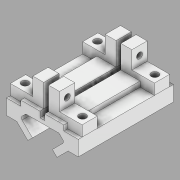
# Autodesk Inventor part: carriage
Saved by Autodesk Inventor 2020 (Build 240168000, 168)
## iProperties
Created: 2021-04-01
Part Number: carriage
Material: ABS Plastic
Document SubType Name: Modeling
Designer: griss
Density: 1.06 g/cm^3
Appearance: Smooth - White
Mass: 192.23 g
Surface Area: 415.711 cm^2
Volume: 181.35 cm^3
Author: griss
Autodesk Inventor part; units mm, degrees
sketch "Sketch1" plane through (0, 0, 0) normal (0, 0, 1) x (1, 0, 0)
  line L0 (0, 17.9605) -> (17.9605, 0) construction
  line L1 (17.9605, 0) -> (0, -17.9605) construction
  line L2 (0, -17.9605) -> (-17.9605, 0) construction
  line L3 (-17.9605, 0) -> (0, 17.9605) construction
  line L4 (0, 17.9605) -> (0, -17.9605) construction
  line L5 (17.9605, 0) -> (-17.9605, 0) construction
  line L6 (0, -30.115) -> (0, 54.9665) projected
  line L7 (-27.2882, 23.4644) -> (-11.7319, 7.908) construction
  line L8 (-11.7319, 7.908) -> (-6.7821, 12.8578) construction
  line L9 (-6.7821, 12.8578) -> (-22.3385, 28.4141) construction
  line L10 (-27.2882, 23.4644) -> (-22.3385, 28.4141) construction
  line L11 (27.2882, 23.4644) -> (11.7319, 7.908) construction
  line L12 (11.7319, 7.908) -> (6.7821, 12.8578) construction
  line L13 (6.7821, 12.8578) -> (22.3385, 28.4141) construction
  line L14 (27.2882, 23.4644) -> (22.3385, 28.4141) construction
  line L15 (-13.3307, 6.837) -> (-29.3711, 22.8773)
  line L16 (-29.3711, 22.8773) -> (-22.2034, 30.045)
  line L17 (-22.2034, 30.045) -> (0, 30.045)
  line L18 (-47.8625, 35.7423) -> (-28.7516, 35.7423)
  line L19 (-28.7516, 35.7423) -> (-28.7516, 42.812)
  line L20 (-28.7516, 42.812) -> (0, 42.812)
  line L21 (-47.8625, 15.4627) -> (-47.8625, 35.7423)
  line L22 (-47.8625, 15.4627) -> (-34.2195, 15.4627)
  line L23 (-34.2195, 15.4627) -> (-19.4622, 0.7055)
  line L24 (-19.4622, 0.7055) -> (-13.3307, 6.837)
  line L25 (13.3307, 6.837) -> (29.3711, 22.8773)
  line L26 (29.3711, 22.8773) -> (22.2034, 30.045)
  line L27 (22.2034, 30.045) -> (0, 30.045)
  line L28 (47.8625, 35.7423) -> (28.7516, 35.7423)
  line L29 (28.7516, 35.7423) -> (28.7516, 42.812)
  line L30 (28.7516, 42.812) -> (0, 42.812)
  line L31 (47.8625, 15.4627) -> (47.8625, 35.7423)
  line L32 (47.8625, 15.4627) -> (34.2195, 15.4627)
  line L33 (34.2195, 15.4627) -> (19.4622, 0.7055)
  line L34 (19.4622, 0.7055) -> (13.3307, 6.837)
  point P0 (0, 0)
  point P1 (0, 0)
  point P2 (0, 0)
  point P3 (0, 0)
  dimension "d2" = 25.4
  dimension "d3" = 25.4
  dimension "d6" = 22
  dimension "d14" = 7
  constraints: 68 end point, 14 horizontal alignment, 6 perpendicular, 4 midpoint, 3 horizontal, 2 coincident, 2 parallel, 1 vertical, 3 other
  measures "d2" distance of L1.end L2.end
  measures "d3" distance of L0.end L1.end
  measures "d6" distance of L8.end L9.end
  measures "d14" distance of L7.end L8.end
extrude "Carriage Frame" add sketch "Sketch1" along normal mid plane 127
fillet "Fillet1" radius 3.175 4 edges at (-29.3711, 22.8773, 0) (-22.2034, 30.045, 0) (22.2034, 30.045, 0) (29.3711, 22.8773, 0)
sketch "Sketch7" plane through (-47.8625, 35.7423, -63.5) normal (0, 1, 0) x (1, 0, 0)
  line L0 (19.1109, 0) -> (76.6141, 0) projected
  line L1 (19.1109, 0) -> (19.1109, -127) projected
  line L2 (76.6141, -127) -> (19.1109, -127) projected
  line L3 (76.6141, 0) -> (76.6141, -127) projected
  line L4 (0, 0) -> (19.1109, 0) projected
  line L5 (0, 0) -> (0, -127) projected
  line L6 (19.1109, -127) -> (0, -127) projected
  line L7 (19.1109, 0) -> (19.1109, -127) projected
  line L8 (76.6141, 0) -> (95.725, 0) projected
  line L9 (76.6141, 0) -> (76.6141, -127) projected
  line L10 (95.725, -127) -> (76.6141, -127) projected
  line L11 (95.725, -127) -> (95.725, 0) projected
  line L12 (19.1109, -63.5) -> (76.6141, -63.5) construction
  line L13 (47.8625, -63.5) -> (47.8625, -63.5) construction
  line L14 (16.8262, -19.4378) -> (9.5554, -23.6355)
  line L15 (9.5554, -23.6355) -> (2.2847, -19.4378)
  line L16 (2.2847, -19.4378) -> (2.2847, -11.0422)
  line L17 (2.2847, -11.0422) -> (9.5554, -6.8445)
  line L18 (9.5554, -6.8445) -> (16.8262, -11.0422)
  line L19 (16.8262, -11.0422) -> (16.8262, -19.4378)
  line L20 (78.8988, -19.4378) -> (86.1695, -23.6355)
  line L21 (86.1695, -23.6355) -> (93.4403, -19.4378)
  line L22 (93.4403, -19.4378) -> (93.4403, -11.0422)
  line L23 (93.4403, -11.0422) -> (86.1695, -6.8445)
  line L24 (86.1695, -6.8445) -> (78.8988, -11.0422)
  line L25 (78.8988, -11.0422) -> (78.8988, -19.4378)
  line L26 (16.8262, -107.5622) -> (9.5554, -103.3645)
  line L27 (9.5554, -103.3645) -> (2.2847, -107.5622)
  line L28 (2.2847, -107.5622) -> (2.2847, -115.9578)
  line L29 (2.2847, -115.9578) -> (9.5554, -120.1555)
  line L30 (9.5554, -120.1555) -> (16.8262, -115.9578)
  line L31 (16.8262, -115.9578) -> (16.8262, -107.5622)
  line L32 (78.8988, -115.9578) -> (78.8988, -107.5622)
  line L33 (86.1695, -120.1555) -> (78.8988, -115.9578)
  line L34 (78.8988, -107.5622) -> (86.1695, -103.3645)
  line L35 (93.4403, -115.9578) -> (86.1695, -120.1555)
  line L36 (93.4403, -107.5622) -> (93.4403, -115.9578)
  line L37 (86.1695, -103.3645) -> (93.4403, -107.5622)
  circle A0 centre (9.5554, -15.24) radius 4.8006
  circle A1 centre (86.1695, -15.24) radius 4.8006
  circle A2 centre (9.5554, -111.76) radius 4.8006
  circle A3 centre (86.1695, -111.76) radius 4.8006
  point P0 (9.5554, 0)
  dimension "d61" = 15.24
  dimension "d78" = 14.5415
  dimension "d79" = 9.6012
  constraints: 52 end point, 27 symmetric about line, 5 coincident, 4 centre point, 4 midpoint, 1 vertical, 1 vertical alignment, 16 other
  measures "d61" distance from line of L4 point (9.555, -15.24)
  measures "d78" distance between parallel lines of L19 L16
  measures "d79" diameter of A0
extrude "Carriage Screw" cut sketch "Sketch7" against normal through all contours A0 | A1 | A2 | A3
extrude "Carriage Screw Insert" cut sketch "Sketch7" against normal blind 6.35 contours L14 L15 L16 L17 L18 L19 | L25 L24 L23 L22 L21 L20 | L31 L30 L29 L28 L27 L26 | L32 L34 L37 L36 L35 L33 | A3
sketch "Ball Bearings" plane through (-13.3307, 6.837, -63.5) normal (0.7071, 0.7071, 0) x (-0.7071, 0.7071, 0)
  line L0 (19.5095, 127) -> (19.5095, 0) projected
  line L1 (0, 127) -> (19.5095, 127) projected
  line L2 (0, 0) -> (0, 127) projected
  line L3 (19.5095, 0) -> (0, 0) projected
  circle A0 centre (7.62, 96.52) radius 4
  line L4 (19.5095, 63.5) -> (0, 63.5) construction
  circle A1 centre (7.62, 30.48) radius 4
  point P0 (-14.2607, 63.5)
  dimension "d94" = 8
  dimension "d106" = 33.02
  dimension "d107" = 7.62
  constraints: 2 centre point, 2 end point, 2 midpoint, 1 symmetric about line, 1 other
  measures "d94" diameter of A0
  measures "d106" distance from line of L4 A0.centre
  measures "d107" distance from line of L2 A0.centre
ref_plane "Carriage Mid Plane" through (0, 15.4627, -63.5) normal (-1, 0, 0) x (0, 0, 1)
extrude "Ball Bearing Hole" cut sketch "Ball Bearings" against normal up to surface (8.6713 mm away) contours A0 | A1
mirror "Mirror4" about plane through (0, 15.4627, -63.5) normal (-1, 0, 0) of "Ball Bearing Hole"
sketch "Sketch13" plane through (0, 0, 63.5) normal (0, 0, 1) x (1, 0, 0)
  line L0 (47.8625, 35.7423) -> (28.7516, 35.7423) projected
  line L1 (28.7516, 35.7423) -> (28.7516, 42.812) projected
  line L2 (28.7516, 42.812) -> (-28.7516, 42.812) projected
  line L3 (-28.7516, 42.812) -> (-28.7516, 35.7423) projected
  line L4 (-28.7516, 35.7423) -> (-47.8625, 35.7423) projected
  line L5 (-47.8625, 35.7423) -> (-47.8625, 15.4627) projected
  line L6 (-47.8625, 15.4627) -> (-34.2195, 15.4627) projected
  line L7 (-34.2195, 15.4627) -> (-19.4622, 0.7055) projected
  line L8 (-19.4622, 0.7055) -> (-13.3307, 6.837) projected
  line L9 (-13.3307, 6.837) -> (-27.126, 20.6323) projected
  arc A0 (-27.126, 25.1224) -> (-27.126, 20.6323) centre (-24.8809, 22.8773) ccw projected
  line L10 (-27.126, 25.1224) -> (-23.1333, 29.1151) projected
  arc A1 (-20.8883, 30.045) -> (-23.1333, 29.1151) centre (-20.8883, 26.87) ccw projected
  line L11 (-20.8883, 30.045) -> (20.8883, 30.045) projected
  arc A2 (23.1333, 29.1151) -> (20.8883, 30.045) centre (20.8883, 26.87) ccw projected
  line L12 (23.1333, 29.1151) -> (27.126, 25.1224) projected
  arc A3 (27.126, 20.6323) -> (27.126, 25.1224) centre (24.8809, 22.8773) ccw projected
  line L13 (27.126, 20.6323) -> (13.3307, 6.837) projected
  line L14 (13.3307, 6.837) -> (19.4622, 0.7055) projected
  line L15 (19.4622, 0.7055) -> (34.2195, 15.4627) projected
  line L16 (34.2195, 15.4627) -> (47.8625, 15.4627) projected
  line L17 (47.8625, 15.4627) -> (47.8625, 35.7423) projected
  line L18 (-3.175, 42.812) -> (3.175, 42.812)
  line L19 (3.175, 42.812) -> (3.175, 35.1375)
  line L20 (3.175, 35.1375) -> (-3.175, 35.1375)
  line L21 (-3.175, 35.1375) -> (-3.175, 42.812)
  point P0 (0, 0)
  point P1 (0, 42.812)
  point P2 (0, 42.812)
  dimension "d112" = 6.35
  constraints: 8 end point, 2 midpoint, 2 parallel, 1 coincident, 1 horizontal, 1 perpendicular, 1 point on line
  measures "d112" distance of L19.end L20.end
extrude "Extrusion11" cut sketch "Sketch13" against normal up to surface (127 mm away) contours L19 L20 L21 L2
ref_plane "Work Plane3" through (0, 0, 48.26) normal (0, 0, 1) x (1, 0, 0)
sketch "Sketch15" plane through (0, 0, 48.26) normal (0, 0, 1) x (1, 0, 0)
  line L0 (-3.175, 35.1375) -> (-3.175, 42.812) projected
  line L1 (-3.175, 42.812) -> (-28.7516, 42.812) projected
  line L2 (-28.7516, 42.812) -> (-28.7516, 35.7423) projected
  line L3 (-28.7516, 35.7423) -> (-47.8625, 35.7423) projected
  line L4 (-47.8625, 35.7423) -> (-47.8625, 15.4627) projected
  line L5 (-47.8625, 15.4627) -> (-34.2195, 15.4627) projected
  line L6 (-34.2195, 15.4627) -> (-19.4622, 0.7055) projected
  line L7 (-19.4622, 0.7055) -> (-13.3307, 6.837) projected
  line L8 (-13.3307, 6.837) -> (-27.126, 20.6323) projected
  arc A0 (-27.126, 25.1224) -> (-27.126, 20.6323) centre (-24.8809, 22.8773) ccw projected
  line L9 (-27.126, 25.1224) -> (-23.1333, 29.1151) projected
  arc A1 (-20.8883, 30.045) -> (-23.1333, 29.1151) centre (-20.8883, 26.87) ccw projected
  line L10 (-20.8883, 30.045) -> (20.8883, 30.045) projected
  arc A2 (23.1333, 29.1151) -> (20.8883, 30.045) centre (20.8883, 26.87) ccw projected
  line L11 (23.1333, 29.1151) -> (27.126, 25.1224) projected
  arc A3 (27.126, 20.6323) -> (27.126, 25.1224) centre (24.8809, 22.8773) ccw projected
  line L12 (27.126, 20.6323) -> (13.3307, 6.837) projected
  line L13 (13.3307, 6.837) -> (19.4622, 0.7055) projected
  line L14 (19.4622, 0.7055) -> (34.2195, 15.4627) projected
  line L15 (34.2195, 15.4627) -> (47.8625, 15.4627) projected
  line L16 (47.8625, 15.4627) -> (47.8625, 35.7423) projected
  line L17 (47.8625, 35.7423) -> (28.7516, 35.7423) projected
  line L18 (28.7516, 35.7423) -> (28.7516, 42.812) projected
  line L19 (28.7516, 42.812) -> (3.175, 42.812) projected
  line L20 (3.175, 42.812) -> (3.175, 35.1375) projected
  line L21 (3.175, 35.1375) -> (-3.175, 35.1375) projected
  line L22 (-3.175, 42.812) -> (-3.175, 80.5116) construction
  line L23 (-3.175, 80.5116) -> (3.175, 80.5116) construction
  line L24 (3.175, 42.812) -> (3.175, 80.5116) construction
  line L25 (-47.8625, 35.7423) -> (-47.8625, 49.9547)
  line L26 (-47.8625, 49.9547) -> (-17.7931, 49.9547)
  line L27 (-17.7931, 49.9547) -> (-17.7931, 73.4726)
  line L28 (-17.7931, 73.4726) -> (-3.175, 73.4726)
  line L29 (-3.175, 73.4726) -> (-3.175, 42.812)
  line L30 (-28.7516, 42.812) -> (-28.7516, 35.7423)
  point P0 (0, 0)
  constraints: 18 end point, 4 perpendicular, 3 vertical, 2 collinear, 1 point on line
extrude "Extrusion12" add sketch "Sketch15" along normal mid plane 20.32 separate body contours L1 L2 L3 L25 L26 L27 L28 L29
sketch "Sketch16" plane through (-47.8625, 49.9547, 58.42) normal (0, 1, 0) x (1, 0, 0)
  circle A0 centre (9.5554, 10.16) radius 4.8006 projected
  point P0 (47.8625, 58.42)
extrude "Extrusion13" cut sketch "Sketch16" against normal through all bodies 2
sketch "Sketch17" plane through (-17.7931, 49.9547, 58.42) normal (-1, 0, 0) x (0, 0, 1)
  line L0 (-20.32, 0) -> (0, 0) projected
  line L1 (0, 23.5178) -> (0, 0) projected
  line L2 (-20.32, 23.5178) -> (0, 23.5178) projected
  line L3 (-20.32, 0) -> (-20.32, 23.5178) projected
  circle A0 centre (-10.16, 11.7589) radius 4
  point P0 (-58.42, -49.9547)
  point P1 (-10.16, 23.5178)
  point P2 (0, 11.7589)
  dimension "d122" = 8
  constraints: 2 midpoint, 1 centre point, 1 horizontal alignment, 1 vertical alignment
  measures "d122" diameter of A0
extrude "Extrusion14" cut sketch "Sketch17" against normal through all contours A0 bodies 2
ref_plane "Work Plane4" through (0, 15.4627, 63.5) normal (-1, 0, 0) x (0, 0, 1)
ref_plane "Work Plane5" through (0, 0, 0) normal (0, 0, -1) x (-1, 0, 0)
mirror "Mirror5" about plane through (0, 15.4627, 63.5) normal (-1, 0, 0) bodies 2
mirror "Mirror6" about plane through (0, 0, 0) normal (0, 0, -1) bodies 2
equation "\"carriage_length\" = 127"
equation "\"ball_bearing_diam\" = 22"
equation "\"ball_bearing_hole\" = 8"
equation "\"d92\" = 8"
body "Solid2"
body "Solid3"
